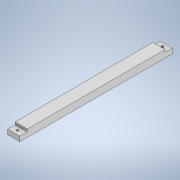
# Autodesk Inventor part: horiz_bar
Saved by Autodesk Inventor 2020 (Build 240168000, 168)
## iProperties
Created: 2022-06-20
Part Number: horiz_bar
Material: 일반
Document SubType Name: Modeling
Designer: samsung
Density: 1 g/cm^3
Appearance: 기본값
Author: samsung
Autodesk Inventor part; units mm, degrees
ref_plane "YZ Plane" through (0, 0, 0) normal (1, 0, 0) x (0, 1, 0)
ref_plane "XZ Plane" through (0, 0, 0) normal (0, 1, 0) x (-1, 0, 0)
ref_plane "XY Plane" through (0, 0, 0) normal (0, 0, 1) x (1, 0, 0)
sketch "스케치1" plane through (0, 0, 0) normal (1, 0, 0) x (0, 1, 0)
  line L0 (-7.5, -154.4285) -> (-7.5, 154.4285)
  line L1 (7.5, 154.4285) -> (7.5, -154.4285)
  line L2 (7.5, -154.4285) -> (-7.5, 154.4285) construction
  line L3 (-7.5, -154.4285) -> (7.5, 154.4285) construction
  line L4 (2.5, 140.5) -> (7.5, 140.5)
  line L5 (7.5, 140.5) -> (7.5, 154.4285)
  line L6 (2.5, -140.5) -> (7.5, -140.5)
  line L7 (7.5, -140.5) -> (7.5, -154.4285)
  line L8 (-7.5, -155.5) -> (-7.5, 155.5)
  line L9 (-7.5, 155.5) -> (7.5, 155.5)
  line L10 (7.5, 155.5) -> (7.5, -155.5)
  line L11 (7.5, -155.5) -> (-7.5, -155.5)
  line L12 (-7.5, -155.5) -> (7.5, 155.5) construction
  line L13 (-7.5, 155.5) -> (7.5, -155.5) construction
  line L14 (2.5, 140.5) -> (2.5, 155.5)
  line L15 (2.5, -140.5) -> (2.5, -155.5)
  point P0 (0, 0)
  point P1 (7.5, -140.5)
  point P2 (7.5, 140.5)
  dimension "d1" = 308.857
  dimension "d2" = 5
  dimension "d14" = 311
  dimension "d15" = 15
  dimension "d25" = 15
  dimension "d26" = 15
  dimension "d27" = 5
  constraints: 32 end point, 4 midpoint, 3 parallel, 2 perpendicular, 2 point on line, 2 vertical
  measures "d1" distance of L0.start L0.end
  measures "d2" distance of L4.end L4.start
  measures "d14" distance of L8.start L8.end
  measures "d15" distance of L8.end L9.end
  measures "d25" distance of L4.start L14.end
  measures "d26" distance of L6.start L15.end
  measures "d27" distance of L6.start L6.end
extrude "돌출1" add sketch "스케치1" along normal blind 25 contours L0 L8 L9 L14 L4 L1 L6 L15 L11
sketch "스케치3" plane through (0, -7.5, -155.5) normal (0, -1, 0) x (1, 0, 0)
  line L0 (0, 311) -> (0, 0) projected
  line L1 (0, 0) -> (25, 0) projected
  line L2 (25, 311) -> (25, 0) projected
  line L3 (0, 311) -> (25, 311) projected
  line L4 (0, 311) -> (0, 0) projected
  line L5 (0, 296) -> (25, 296) projected
  line L6 (25, 296) -> (0, 296)
  line L7 (0, 296) -> (0, 311)
  line L8 (0, 311) -> (25, 311)
  line L9 (25, 311) -> (25, 296)
  line L10 (0, 15) -> (25, 15) projected
  line L11 (25, 311) -> (25, 0) projected
  line L12 (25, 0) -> (0, 0)
  line L13 (0, 0) -> (0, 15)
  line L14 (0, 15) -> (25, 15)
  line L15 (25, 15) -> (25, 0)
  point P0 (0, 155.5)
  point P1 (12.5, 303.5)
  point P2 (12.5, 7.5)
  constraints: 16 end point, 4 parallel, 2 horizontal, 2 perpendicular
hole "구멍3" at (12.5, -7.5, 148) at (12.5, -7.5, -148) direction (0, 1, 0) diameter 4.134 end through all counterbore diameter 9 counterbore depth 5 thread size "M5x0.8" class "6H" standard "ISO Metric profile"
